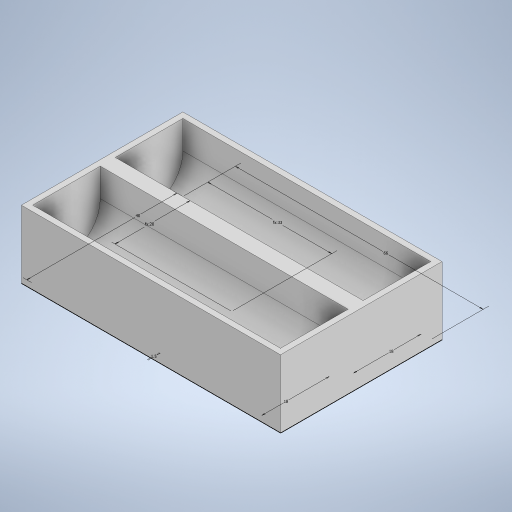
# Autodesk Inventor part: battery rack
Saved by Autodesk Inventor 2023 (Build 270158000, 158)
## iProperties
Created: 2023-03-17
Part Number: battery rack
Material: Generic
Document SubType Name: Modeling
Designer: user
Density: 1 g/cm^3
Appearance: Default
Author: user
Autodesk Inventor part; units mm, degrees
ref_plane "YZ Plane" through (0, 0, 0) normal (1, 0, 0) x (0, 1, 0)
ref_plane "XZ Plane" through (0, 0, 0) normal (0, 1, 0) x (-1, 0, 0)
ref_plane "XY Plane" through (0, 0, 0) normal (0, 0, 1) x (1, 0, 0)
sketch "Sketch1" plane through (0, 0, 0) normal (0, 1, 0) x (-1, 0, 0)
  line L0 (33, 20) -> (-33, 20)
  line L1 (-33, 20) -> (-33, -20)
  line L2 (-33, -20) -> (33, -20)
  line L3 (33, -20) -> (33, 20)
  line L4 (33, 2) -> (-33, 2)
  line L5 (33, -2) -> (-33, -2)
  line L6 (-34.5, 21.5) -> (34.5, 21.5)
  line L7 (34.5, 21.5) -> (34.5, -21.5)
  line L8 (34.5, -21.5) -> (-34.5, -21.5)
  line L9 (-34.5, -21.5) -> (-34.5, 21.5)
  point P0 (0, 0)
  dimension "d0" = 66
  dimension "d1" = 33
  dimension "d2" = 40
  dimension "d3" = 20
  dimension "d4" = 18
  dimension "d5" = 18
  dimension "d6" = 1.5
  constraints: 20 end point, 4 parallel, 4 perpendicular, 4 point on line, 1 horizontal, 3 other
  measures "d0" distance between parallel lines of L1 L3
  measures "d1" distance from line of point (0, 0) L3
  measures "d2" distance of L2.end L0.start
  measures "d3" distance from line of point (0, 0) L2
  measures "d4" distance between parallel lines of L5 L2
  measures "d5" distance between parallel lines of L0 L4
  measures "d6" distance between parallel lines of L0 L6
extrude "Extrusion1" add sketch "Sketch1" along normal blind 1.5 contours L3 L4 L1 L0 | L3 L5 L1 L4 | L3 L2 L1 L5 | L6 L7 L8 L9
sketch "Sketch2" plane through (0, 1.5, 0) normal (0, 1, 0) x (1, 0, 0)
  point P0 (0, 0)
extrude "Extrusion2" add sketch "Sketch1" along normal blind 18 contours L3 L5 L1 L4 | L6 L7 L8 L9
fillet "Fillet1" radius 9 4 edges at (0, 1.5, 2) (0, 1.5, 20) (0, 1.5, -2) (0, 1.5, -20)
equation "\"d1\" = 0.5 * d0"
equation "\"d3\" = 0.5 * d2"
body "Solid1"
